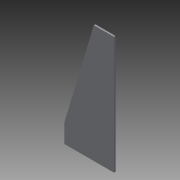
# Autodesk Inventor part: FRAME SIDE
Saved by Autodesk Inventor 2013 (Build 170138000, 138)
## iProperties
Created: 2014-03-04
Part Number: FRAME SIDE
Material: Generic
Document SubType Name: Modeling
Designer: employee
Density: 1 g/cm^3
Author: employee
Autodesk Inventor part; units mm, degrees
ref_plane "YZ Plane" through (0, 0, 0) normal (1, 0, 0) x (0, 1, 0)
ref_plane "XZ Plane" through (0, 0, 0) normal (0, 1, 0) x (-1, 0, 0)
ref_plane "XY Plane" through (0, 0, 0) normal (0, 0, 1) x (1, 0, 0)
ref_plane "Work Plane1" through (0, 0, 0) normal (0, 0, 1) x (1, 0, 0)
sketch "Sketch2" plane through (0, 0, 0) normal (0, 0, 1) x (1, 0, 0)
  line L0 (0, 0) -> (100, 0) projected
  line L1 (0, 6.477) -> (100, 6.477) projected
  line L2 (150, 402.5) -> (150, 427.5) projected
  line L3 (156.477, 427.5) -> (156.477, 402.5) projected
  line L4 (150, 427.5) -> (156.477, 427.5) projected
  line L5 (150, -75) -> (-50, -75)
  line L6 (-50, -75) -> (-50, 0)
  line L7 (-50, 0) -> (150, 0)
  line L8 (150, 0) -> (150, -75)
  line L9 (150, 427.5) -> (75, 427.5)
  line L10 (75, 427.5) -> (-50, 6.477)
  line L11 (150, 6.477) -> (150, 427.5)
  line L12 (150, 402.5) -> (156.477, 402.5) projected
  line L13 (156.477, 427.5) -> (150, 427.5)
  line L14 (150, 427.5) -> (150, -75)
  line L15 (150, -75) -> (156.477, -75)
  line L16 (156.477, -75) -> (156.477, 427.5)
  line L17 (-50, 6.477) -> (-50, 0)
  line L18 (-50, 0) -> (150, 0)
  line L19 (150, 0) -> (150, 427.5)
  line L20 (100, 0) -> (100, 6.477) projected
  line L21 (0, 6.477) -> (0, 0) projected
  dimension "d3" = 75
  constraints: 28 end point, 6 parallel, 4 perpendicular, 2 horizontal, 1 collinear
  measures "d3" distance of L2.end L9.end
extrude "Extrusion2" add sketch "Sketch2" along normal blind 6.477
sketch "Sketch5" plane through (156.477, -75, 0) normal (1, 0, 0) x (0, 0, -1)
  line L0 (0, 0) -> (0, 502.5) projected
  line L1 (0, 502.5) -> (-6.477, 502.5) projected
  line L2 (-6.477, 0) -> (-6.477, 502.5) projected
  line L3 (0, 0) -> (-6.477, 0) projected
  point P0 (0, 75)
  point P1 (0, 477.5)
  point P2 (-6.477, 477.5)
extrude "Extrusion5" add sketch "Sketch5" along normal blind 5
sketch "Sketch6" plane through (0, 0, 6.477) normal (0, 0, 1) x (1, 0, 0)
  line L0 (-50, -75) -> (161.477, -75) projected
  arc A0 (136.477, -75) -> (-25, -75) centre (55.7385, -284.7902) ccw
  point P0 (0, 0)
  point P1 (55.7385, -60)
  point P2 (55.7385, -75)
  point P3 (150, -75)
  point P4 (156.477, -75)
  dimension "d14" = 25
  dimension "d15" = 15
  constraints: 3 point on circle, 2 point on line, 1 centre point, 1 midpoint, 1 vertical alignment
  measures "d14" distance of A0.end L0.start
  measures "d15" distance of point (55.739, -60) point (55.739, -75)
extrude "Extrusion6" cut sketch "Sketch6" against normal through all
sketch "Sketch7" plane through (0, 0, 6.477) normal (0, 0, 1) x (1, 0, 0)
  line L0 (-45, -25) -> (-45, -50) projected
  line L1 (-45, -50) -> (-38.523, -50) projected
  line L2 (-38.523, -25) -> (-38.523, -50) projected
  line L3 (-45, -25) -> (-38.523, -25) projected
  line L4 (150, -50) -> (150, -25) projected
  line L5 (156.477, -50) -> (150, -50) projected
  line L6 (156.477, -25) -> (156.477, -50) projected
  line L7 (156.477, -25) -> (150, -25) projected
  line L8 (150, 92.5) -> (150, 117.5) projected
  line L9 (156.477, 92.5) -> (150, 92.5) projected
  line L10 (156.477, 117.5) -> (156.477, 92.5) projected
  line L11 (156.477, 117.5) -> (150, 117.5) projected
  line L12 (150, 235) -> (150, 260) projected
  line L13 (156.477, 235) -> (150, 235) projected
  line L14 (156.477, 260) -> (156.477, 235) projected
  line L15 (156.477, 260) -> (150, 260) projected
  line L16 (150, 377.5) -> (150, 402.5) projected
  line L17 (156.477, 377.5) -> (150, 377.5) projected
  line L18 (156.477, 402.5) -> (156.477, 377.5) projected
  line L19 (156.477, 402.5) -> (150, 402.5) projected
  line L20 (125, 422.5) -> (100, 422.5) projected
  line L21 (100, 422.5) -> (100, 416.023) projected
  line L22 (125, 416.023) -> (100, 416.023) projected
  line L23 (125, 422.5) -> (125, 416.023) projected
  line L24 (0, 0) -> (-25, 0) projected
  line L25 (0, 6.477) -> (0, 0) projected
  line L26 (-25, 6.477) -> (0, 6.477) projected
  line L27 (-25, 6.477) -> (-25, 0) projected
  line L28 (125, 0) -> (100, 0) projected
  line L29 (125, 6.477) -> (125, 0) projected
  line L30 (100, 6.477) -> (125, 6.477) projected
  line L31 (100, 6.477) -> (100, 0) projected
extrude "Extrusion7" cut sketch "Sketch7" against normal through all
sketch "Sketch8" plane through (0, 0, 6.477) normal (0, 0, 1) x (1, 0, 0)
  line L0 (-25, 0) -> (-25, 6.477) projected
  line L1 (-25, 6.477) -> (0, 6.477) projected
  line L2 (-45, -50) -> (-45, -25) projected
  line L3 (-45, -25) -> (-38.523, -25) projected
  line L4 (100, 416.023) -> (100, 422.5) projected
  line L5 (125, 416.023) -> (100, 416.023) projected
  line L6 (100, 0) -> (100, 6.477) projected
  line L7 (100, 6.477) -> (125, 6.477) projected
  line L8 (-47.5, -35.5) -> (-36.023, -35.5)
  line L9 (-36.023, -35.5) -> (-36.023, -39.5)
  line L10 (-36.023, -39.5) -> (-47.5, -39.5)
  line L11 (-47.5, -39.5) -> (-47.5, -35.5)
  line L12 (-47.5, -35.5) -> (-49, -35.5)
  line L13 (-49, -35.5) -> (-49, -39.5)
  line L14 (-49, -39.5) -> (-47.5, -39.5)
  line L15 (-47.5, -39.5) -> (-47.5, -35.5)
  line L16 (-36.023, -35.5) -> (-34.523, -35.5)
  line L17 (-34.523, -35.5) -> (-34.523, -39.5)
  line L18 (-34.523, -39.5) -> (-36.023, -39.5)
  line L19 (-36.023, -39.5) -> (-36.023, -35.5)
  line L20 (147.5, -35.5) -> (158.977, -35.5)
  line L21 (158.977, -35.5) -> (158.977, -39.5)
  line L22 (158.977, -39.5) -> (147.5, -39.5)
  line L23 (147.5, -39.5) -> (147.5, -35.5)
  line L24 (147.5, -35.5) -> (146, -35.5)
  line L25 (146, -35.5) -> (146, -39.5)
  line L26 (146, -39.5) -> (147.5, -39.5)
  line L27 (147.5, -39.5) -> (147.5, -35.5)
  line L28 (158.977, -35.5) -> (160.477, -35.5)
  line L29 (160.477, -35.5) -> (160.477, -39.5)
  line L30 (160.477, -39.5) -> (158.977, -39.5)
  line L31 (158.977, -39.5) -> (158.977, -35.5)
  line L32 (147.5, 107) -> (158.977, 107)
  line L33 (158.977, 107) -> (158.977, 103)
  line L34 (158.977, 103) -> (147.5, 103)
  line L35 (147.5, 103) -> (147.5, 107)
  line L36 (147.5, 107) -> (146, 107)
  line L37 (146, 107) -> (146, 103)
  line L38 (146, 103) -> (147.5, 103)
  line L39 (147.5, 103) -> (147.5, 107)
  line L40 (158.977, 107) -> (160.477, 107)
  line L41 (160.477, 107) -> (160.477, 103)
  line L42 (160.477, 103) -> (158.977, 103)
  line L43 (158.977, 103) -> (158.977, 107)
  line L44 (147.5, 249.5) -> (158.977, 249.5)
  line L45 (158.977, 249.5) -> (158.977, 245.5)
  line L46 (158.977, 245.5) -> (147.5, 245.5)
  line L47 (147.5, 245.5) -> (147.5, 249.5)
  line L48 (147.5, 249.5) -> (146, 249.5)
  line L49 (146, 249.5) -> (146, 245.5)
  line L50 (146, 245.5) -> (147.5, 245.5)
  line L51 (147.5, 245.5) -> (147.5, 249.5)
  line L52 (158.977, 249.5) -> (160.477, 249.5)
  line L53 (160.477, 249.5) -> (160.477, 245.5)
  line L54 (160.477, 245.5) -> (158.977, 245.5)
  line L55 (158.977, 245.5) -> (158.977, 249.5)
  line L56 (147.5, 392) -> (158.977, 392)
  line L57 (158.977, 392) -> (158.977, 388)
  line L58 (158.977, 388) -> (147.5, 388)
  line L59 (147.5, 388) -> (147.5, 392)
  line L60 (147.5, 392) -> (146, 392)
  line L61 (146, 392) -> (146, 388)
  line L62 (146, 388) -> (147.5, 388)
  line L63 (147.5, 388) -> (147.5, 392)
  line L64 (158.977, 392) -> (160.477, 392)
  line L65 (160.477, 392) -> (160.477, 388)
  line L66 (160.477, 388) -> (158.977, 388)
  line L67 (158.977, 388) -> (158.977, 392)
  line L68 (110.5, 413.523) -> (110.5, 425)
  line L69 (110.5, 425) -> (114.5, 425)
  line L70 (114.5, 425) -> (114.5, 413.523)
  line L71 (114.5, 413.523) -> (110.5, 413.523)
  line L72 (110.5, 413.523) -> (110.5, 412.023)
  line L73 (110.5, 412.023) -> (114.5, 412.023)
  line L74 (114.5, 412.023) -> (114.5, 413.523)
  line L75 (114.5, 413.523) -> (110.5, 413.523)
  line L76 (110.5, 425) -> (110.5, 426.5)
  line L77 (110.5, 426.5) -> (114.5, 426.5)
  line L78 (114.5, 426.5) -> (114.5, 425)
  line L79 (114.5, 425) -> (110.5, 425)
  line L80 (-14.5, -2.5) -> (-14.5, -4)
  line L81 (-10.5, -4) -> (-10.5, -2.5)
  line L82 (-14.5, -4) -> (-10.5, -4)
  line L83 (-14.5, -2.5) -> (-14.5, 8.977)
  line L84 (-14.5, 8.977) -> (-10.5, 8.977)
  line L85 (-10.5, 8.977) -> (-10.5, -2.5)
  line L86 (-10.5, -2.5) -> (-14.5, -2.5)
  line L87 (-14.5, 8.977) -> (-14.5, 10.477)
  line L88 (-14.5, 10.477) -> (-10.5, 10.477)
  line L89 (-10.5, 10.477) -> (-10.5, 8.977)
  line L90 (-10.5, 8.977) -> (-14.5, 8.977)
  line L91 (-10.5, -2.5) -> (-14.5, -2.5)
  line L92 (110.5, -2.5) -> (110.5, -4)
  line L93 (114.5, -4) -> (114.5, -2.5)
  line L94 (110.5, -4) -> (114.5, -4)
  line L95 (110.5, -2.5) -> (110.5, 8.977)
  line L96 (110.5, 8.977) -> (114.5, 8.977)
  line L97 (114.5, 8.977) -> (114.5, -2.5)
  line L98 (114.5, -2.5) -> (110.5, -2.5)
  line L99 (110.5, 8.977) -> (110.5, 10.477)
  line L100 (110.5, 10.477) -> (114.5, 10.477)
  line L101 (114.5, 10.477) -> (114.5, 8.977)
  line L102 (114.5, 8.977) -> (110.5, 8.977)
  line L103 (114.5, -2.5) -> (110.5, -2.5)
  point P0 (-47.5, -37.5)
  point P1 (-45, -37.5)
  point P2 (-41.7615, -35.5)
  point P3 (-41.7615, -25)
  point P4 (147.5, -37.5)
  point P5 (150, -37.5)
  point P6 (153.2385, -35.5)
  point P7 (147.5, 105)
  point P8 (150, 105)
  point P9 (153.2385, 107)
  point P10 (147.5, 247.5)
  point P11 (150, 247.5)
  point P12 (153.2385, 249.5)
  point P13 (147.5, 390)
  point P14 (150, 390)
  point P15 (153.2385, 392)
  point P16 (112.5, 413.523)
  point P17 (112.5, 416.023)
  point P18 (110.5, 419.2615)
  point P19 (100, 419.2615)
  point P20 (112.5, 413.523)
  point P21 (112.5, 416.023)
  point P22 (-12.5, -2.5)
  point P23 (-11.1358, -0.405)
  point P24 (-14.5, 3.2385)
  point P25 (-12.5, -2.5)
  point P26 (-12.5, 0)
  point P27 (112.5, -2.5)
  point P28 (112.5, 0)
  point P29 (110.5, 3.2385)
  point P30 (112.5, -2.5)
  point P31 (112.5, 0)
  point P32 (-12.5, 8.977)
  point P33 (-12.5, 6.477)
  point P34 (-25, 3.2385)
  point P35 (112.5, 8.977)
  point P36 (112.5, 6.477)
  point P37 (100, 3.2385)
  dimension "d20" = 2.5
  dimension "d21" = 1.5
  dimension "d22" = 4
  dimension "d23" = 1.5
  dimension "d24" = 4
  dimension "d25" = 1.5
  dimension "d26" = 4
  dimension "d27" = 1.5
  dimension "d28" = 4
  dimension "d29" = 1.5
  dimension "d30" = 4
  dimension "d31" = 1.5
  dimension "d32" = 4
  dimension "d33" = 2.5
  dimension "d34" = 1.5
  dimension "d35" = 4
  dimension "d36" = 1.5
  dimension "d37" = 4
  dimension "d38" = 2.5
  dimension "d39" = 2.5
  constraints: 192 end point, 48 parallel, 29 midpoint, 24 perpendicular, 15 horizontal, 8 collinear, 8 horizontal alignment, 6 vertical alignment, 3 vertical
  measures "d20" distance between parallel lines of L2 L11
  measures "d21" distance of L13.end L10.end
  measures "d22" distance of L12.end L13.end
  measures "d23" distance of L26.start L26.end
  measures "d24" distance of L24.end L26.start
  measures "d25" distance of L38.start L38.end
  measures "d26" distance of L36.end L38.start
  measures "d27" distance of L50.start L50.end
  measures "d28" distance of L48.end L50.start
  measures "d29" distance of L62.start L62.end
  measures "d30" distance of L60.end L62.start
  measures "d31" distance of L74.start L74.end
  measures "d32" distance of L72.end L74.start
  measures "d33" distance from line of L5 point (112.5, 413.523)
  measures "d34" distance of L81.start L81.end
  measures "d35" distance of L80.end L81.start
  measures "d36" distance of L93.start L93.end
  measures "d37" distance of L92.end L93.start
  measures "d38" distance between parallel lines of L1 L90
  measures "d39" distance from line of L96 point (112.5, 6.477)
extrude "Extrusion8" cut sketch "Sketch8" against normal through all contours L86 L81 L82 L80 | L87 L88 L89 L84 | L9 L16 L17 L18 | L14 L13 L12 L11 | L69 L76 L77 L78 | L74 L73 L72 L71 | L98 L93 L94 L92 | L99 L100 L101 L96 | L23 L26 L25 L24 | L28 L29 L30 L21 | L35 L38 L37 L36 | L40 L41 L42 L33 | L47 L50 L49 L48 | L52 L53 L54 L45 | L59 L62 L61 L60 | L64 L65 L66 L57
sketch "Sketch9" plane through (0, 0, 0) normal (0, 0, -1) x (-1, 0, 0)
  line L0 (0, 6.477) -> (25, 6.477) projected
  line L1 (-150, 260) -> (-150, 235) projected
  circle A0 centre (-25, 156.477) radius 4
  dimension "d42" = 8
  dimension "d44" = 125
  dimension "d45" = 150
  constraints: 1 centre point
  measures "d42" diameter of A0
  measures "d44" distance from line of A0.centre L1
  measures "d45" distance from line of L0 A0.centre
extrude "Extrusion9" cut sketch "Sketch9" against normal through all
sketch "Sketch10" plane through (0, 0, 6.477) normal (0, 0, 1) x (1, 0, 0)
  line L0 (150, 377.5) -> (150, 402.5) projected
  line L1 (125, 416.023) -> (100, 416.023) projected
  line L2 (103, 369.023) -> (103, 411.023)
  line L3 (103, 411.023) -> (145, 411.023)
  line L4 (145, 411.023) -> (145, 369.023)
  line L5 (145, 369.023) -> (103, 369.023)
  circle A0 centre (124, 390.023) radius 11
  line L6 (108.5, 405.523) -> (139.5, 405.523)
  line L7 (139.5, 405.523) -> (139.5, 374.523)
  line L8 (139.5, 374.523) -> (108.5, 374.523)
  line L9 (108.5, 374.523) -> (108.5, 405.523)
  circle A1 centre (108.5, 405.523) radius 1.5
  circle A2 centre (139.5, 405.523) radius 1.5
  circle A3 centre (139.5, 374.523) radius 1.5
  circle A4 centre (108.5, 374.523) radius 1.5
  line L10 (116.5, 349.023) -> (116.5, 324.023)
  arc A5 (116.5, 324.023) -> (131.5, 324.023) centre (124, 324.023) ccw
  line L11 (131.5, 324.023) -> (131.5, 349.023)
  arc A6 (131.5, 349.023) -> (116.5, 349.023) centre (124, 349.023) ccw
  point P0 (124, 405.523)
  dimension "d48" = 5
  dimension "d49" = 5
  dimension "d50" = 42
  dimension "d51" = 22
  dimension "d52" = 31
  dimension "d53" = 3
  dimension "d54" = 20
  dimension "d55" = 25
  dimension "d56" = 15
  constraints: 20 end point, 7 centre point, 6 coincident, 4 point on circle, 4 tangent, 3 equal radius, 2 parallel, 1 horizontal, 1 horizontal alignment, 1 midpoint, 1 vertical alignment, 18 other
  measures "d48" distance between parallel lines of L1 L3
  measures "d49" distance between parallel lines of L0 L4
  measures "d50" distance of L4.end L2.start
  measures "d51" diameter of A0
  measures "d52" distance of L6.start L6.end
  measures "d53" diameter of A1
  measures "d54" distance from line of L5 A6.centre
  measures "d55" distance of L11.start L11.end
  measures "d56" distance between parallel lines of L10 L11
extrude "Extrusion10" cut sketch "Sketch10" against normal through all contours A0 | L9 A1 L6 | L6 A1 L9 | A2 L7 L6 | L6 L7 A2 | A4 L8 L9 | L9 L8 A4 | A3 L8 L7 | L7 L8 A3 | A6 L11 A5 L10
sketch "Sketch4" plane through (0, 0, 6.477) normal (0, 0, 1) x (1, 0, 0)
  line L0 (-50, -75) -> (156.477, -75) projected
  arc A0 (131.477, -75) -> (-25, -75) centre (53.2385, -271.5421) ccw
  point P0 (161.477, -75)
  point P1 (0, 0)
  point P2 (53.2385, -60)
  point P3 (53.2385, -75)
  point P4 (150, -75)
  dimension "d8" = 15
  dimension "d9" = 25
  constraints: 3 point on circle, 2 point on line, 1 centre point, 1 midpoint, 1 vertical alignment
  measures "d8" distance from line of point (53.239, -60) L0
  measures "d9" distance of A0.end L0.start
body "Solid2"
